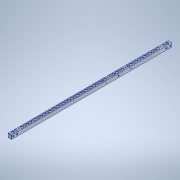
# Autodesk Inventor part: ロボットベース15x15_1
Saved by Autodesk Inventor 2020.3 (Build 243373000, 373)
## iProperties
Created: 2020-07-04
Part Number: ロボットベース15x15_1
Material: アルミニウム 6061
Document SubType Name: Modeling
Designer: totot
Density: 2.7 g/cm^3
Appearance: アルミニウム - フラット
Mass: 89.7951 g
Surface Area: 597.989 cm^2
Volume: 33.2574 cm^3
Author: totot
Autodesk Inventor part; units mm, degrees
ref_plane "YZ Plane" through (0, 0, 0) normal (1, 0, 0) x (0, 1, 0)
ref_plane "XZ Plane" through (0, 0, 0) normal (0, 1, 0) x (-1, 0, 0)
ref_plane "XY Plane" through (0, 0, 0) normal (0, 0, 1) x (1, 0, 0)
sketch "スケッチ1" plane through (0, 0, 0) normal (0, 0, 1) x (1, 0, 0)
  line L0 (0, 0) -> (-15, 0)
  line L1 (-15, 0) -> (-15, -15)
  line L2 (-15, -15) -> (0, -15)
  line L3 (0, -15) -> (0, 0)
  line L4 (-13.8, -1.2) -> (-1.2, -1.2)
  line L5 (-1.2, -1.2) -> (-1.2, -13.8)
  line L6 (-1.2, -13.8) -> (-13.8, -13.8)
  line L7 (-13.8, -13.8) -> (-13.8, -1.2)
  dimension "d0" = 15
  dimension "d1" = 15
  dimension "d2" = 1.2
  dimension "d3" = 1.2
  dimension "d4" = 1.2
  dimension "d5" = 1.2
  constraints: 16 end point, 4 parallel, 2 horizontal, 2 perpendicular
  measures "d0" distance of L2.end L1.end
  measures "d1" distance of L1.end L0.end
  measures "d2" distance between parallel lines of L1 L7
  measures "d3" distance between parallel lines of L4 L0
  measures "d4" distance between parallel lines of L2 L6
  measures "d5" distance between parallel lines of L5 L3
extrude "押し出し1" add sketch "スケッチ1" along normal blind 655
sketch "スケッチ2" plane through (0, -15, 0) normal (1, 0, 0) x (0, 0, -1)
  line L0 (-655, 0) -> (-655, 15) projected
  line L1 (0, 15) -> (-655, 15) projected
  line L2 (0, 0) -> (0, 15) projected
  point P0 (-7.5, 7.5)
  point P1 (-647.5, 7.5)
  dimension "d8" = 7.5
  dimension "d9" = 7.5
  dimension "d10" = 7.5
  dimension "d11" = 7.5
  measures "d8" distance from line of point (-647.5, 7.5) L0
  measures "d9" distance from line of point (-647.5, 7.5) L1
  measures "d10" distance from line of point (-7.5, 7.5) L1
  measures "d11" distance from line of point (-7.5, 7.5) L2
hole "穴1" at (0, -7.5, 7.5) at (0, -7.5, 647.5) direction (-1, 0, 0) diameter 5 end through all
sketch "スケッチ3" plane through (-15, -15, 0) normal (-1, 0, 0) x (0, 0, 1)
  line L0 (0, 0) -> (655, 0) projected
  circle A0 centre (7.5, 7.5) radius 2.5 projected
  circle A1 centre (647.5, 7.5) radius 2.5 projected
  point P0 (0, 15)
  point P1 (22.5, 7.5)
  point P2 (632.5, 7.5)
  dimension "d19" = 7.5
  dimension "d20" = 15
  dimension "d21" = 7.5
  dimension "d22" = 15
  measures "d19" distance from line of point (22.5, 7.5) L0
  measures "d20" distance of point (22.5, 7.5) A0.centre
  measures "d21" distance from line of L0 point (632.5, 7.5)
  measures "d22" distance of point (632.5, 7.5) A1.centre
hole "穴2" at (-15, -7.5, 22.5) at (-15, -7.5, 632.5) direction (1, 0, 0) diameter 3 depth 5 tip angle 118
sketch "スケッチ4" plane through (-1.2, -13.8, 0) normal (-1, 0, 0) x (0, 0, 1)
  circle A0 centre (22.5, 6.3) radius 1.5 projected
  circle A1 centre (632.5, 6.3) radius 1.5 projected
  point P0 (0, 13.8)
  constraints: 2 coincident
hole "穴3" at (-1.2, -7.5, 22.5) at (-1.2, -7.5, 632.5) direction (1, 0, 0) diameter 6 end through all
sketch "スケッチ6" plane through (-15, 0, 0) normal (0, 1, 0) x (1, 0, 0)
  line L0 (15, -655) -> (0, -655) projected
  line L1 (15, 0) -> (15, -655) projected
  line L2 (15, 0) -> (0, 0) projected
  point P0 (7.5, -37.5)
  point P1 (7.5, -617.5)
  dimension "d37" = 37.5
  dimension "d38" = 7.5
  dimension "d39" = 7.5
  dimension "d40" = 37.5
  measures "d37" distance from line of point (7.5, -617.5) L0
  measures "d38" distance from line of point (7.5, -617.5) L1
  measures "d39" distance from line of point (7.5, -37.5) L1
  measures "d40" distance from line of point (7.5, -37.5) L2
hole "穴4" at (-7.5, 0, 37.5) at (-7.5, 0, 617.5) direction (0, -1, 0) diameter 3 end through all
sketch "スケッチ7" plane through (-15, -15, 0) normal (-1, 0, 0) x (0, 0, 1)
  line L0 (0, 15) -> (655, 15) projected
  line L1 (0, 15) -> (0, 0) projected
  point P0 (218.3333, 7.5)
  dimension "d59" = 655
  dimension "d60" = 218.3333
  dimension "d61" = 7.5
  measures "d59" distance of L0.start L0.end
  measures "d60" distance from line of point (218.333, 7.5) L1
  measures "d61" distance from line of point (218.333, 7.5) L0
hole "穴5" at (-15, -7.5, 218.3333) direction (1, 0, 0) diameter 5 end through all
sketch "スケッチ8" plane through (-15, -15, 0) normal (-1, 0, 0) x (0, 0, 1)
  line L0 (0, 15) -> (655, 15) projected
  circle A0 centre (218.3333, 7.5) radius 2.5 projected
  point P0 (167.8333, 7.5)
  point P1 (268.8333, 7.5)
  dimension "d62" = 7.5
  dimension "d63" = 7.5
  dimension "d64" = 101
  dimension "d65" = 50.5
  measures "d62" distance from line of point (167.833, 7.5) L0
  measures "d63" distance from line of point (268.833, 7.5) L0
  measures "d64" distance of point (268.833, 7.5) point (167.833, 7.5)
  measures "d65" distance of point (167.833, 7.5) A0.centre
hole "穴6" at (-15, -7.5, 167.8333) at (-15, -7.5, 268.8333) direction (1, 0, 0) diameter 3 end through all
sketch "スケッチ9" plane through (-15, 0, 0) normal (0, 1, 0) x (1, 0, 0)
  line L0 (15, 0) -> (15, -655) projected
  line L1 (15, 0) -> (0, 0) projected
  point P0 (7.5, -182.8333)
  point P1 (7.5, -253.8333)
  point P2 (9.8445, -218.3333)
  dimension "d73" = 7.5
  dimension "d74" = 7.5
  dimension "d75" = 71
  dimension "d76" = 655
  dimension "d85" = 218.3333
  dimension "d86" = 35.5
  measures "d73" distance from line of point (7.5, -182.833) L0
  measures "d74" distance from line of point (7.5, -253.833) L0
  measures "d75" distance of point (7.5, -182.833) point (7.5, -253.833)
  measures "d76" distance of L0.start L0.end
  measures "d85" distance from line of L1 point (9.844, -218.333)
  measures "d86" vertical distance of point (9.844, -218.333) point (7.5, -253.833)
hole "穴7" at (-7.5, 0, 182.8333) at (-7.5, 0, 253.8333) direction (0, -1, 0) diameter 3 end through all
sketch "スケッチ10" plane through (-15, -15, 0) normal (0, -1, 0) x (1, 0, 0)
  circle A0 centre (7.5, 37.5) radius 1.5 projected
  line L0 (0, 0) -> (15, 0) projected
  line L1 (0, 0) -> (0, 655) projected
  line L2 (0, 655) -> (15, 655) projected
  circle A1 centre (7.5, 182.8333) radius 1.5 projected
  circle A2 centre (7.5, 253.8333) radius 1.5 projected
  circle A3 centre (7.5, 617.5) radius 1.5 projected
  point P0 (7.5, 12.5)
  point P1 (7.5, 25)
  point P2 (7.5, 630)
  point P3 (7.5, 642.5)
  point P4 (7.5, 48.6795)
  point P5 (7.5, 194.6667)
  point P6 (7.5, 206.5)
  point P7 (7.5, 218.3333)
  point P8 (7.5, 230.1667)
  point P9 (7.5, 242)
  point P10 (7.5, 59.859)
  point P11 (7.5, 71.0385)
  point P12 (7.5, 82.2179)
  point P13 (7.5, 93.3974)
  point P14 (7.5, 104.5769)
  point P15 (7.5, 115.7564)
  point P16 (7.5, 126.9359)
  point P17 (7.5, 138.1154)
  point P18 (7.5, 149.2949)
  point P19 (7.5, 160.4744)
  point P20 (7.5, 171.6538)
  point P21 (7.5, 265.1979)
  point P22 (7.5, 276.5625)
  point P23 (7.5, 287.9271)
  point P24 (7.5, 299.2917)
  point P25 (7.5, 310.6562)
  point P26 (7.5, 322.0208)
  point P27 (7.5, 333.3854)
  point P28 (7.5, 344.75)
  point P29 (7.5, 356.1146)
  point P30 (7.5, 367.4792)
  point P31 (7.5, 378.8438)
  point P32 (7.5, 390.2083)
  point P33 (7.5, 401.5729)
  point P34 (7.5, 412.9375)
  point P35 (7.5, 424.3021)
  point P36 (7.5, 435.6667)
  point P37 (7.5, 447.0312)
  point P38 (7.5, 458.3958)
  point P39 (7.5, 469.7604)
  point P40 (7.5, 481.125)
  point P41 (7.5, 492.4896)
  point P42 (7.5, 503.8542)
  point P43 (7.5, 515.2188)
  point P44 (7.5, 526.5833)
  point P45 (7.5, 537.9479)
  point P46 (7.5, 549.3125)
  point P47 (7.5, 560.6771)
  point P48 (7.5, 572.0417)
  point P49 (7.5, 583.4062)
  point P50 (7.5, 594.7708)
  point P51 (7.5, 606.1354)
  dimension "d87" = 37.5
  dimension "d88" = 7.5
  dimension "d89" = 7.5
  dimension "d90" = 12.5
  dimension "d91" = 12.5
  dimension "d92" = 7.5
  dimension "d93" = 7.5
  dimension "d94" = 12.5
  dimension "d95" = 12.5
  dimension "d96" = 7.5
  dimension "d97" = 145.3333
  dimension "d98" = 71
  dimension "d101" = 11.8333
  dimension "d106" = 7.5
  dimension "d107" = 11.8333
  dimension "d108" = 11.1795
  dimension "d111" = 11.1795
  dimension "d116" = 363.6667
  dimension "d117" = 11.3646
  dimension "d118" = 7.5
  dimension "d121" = 11.3646
  constraints: 3 vertical, 45 other
  measures "d87" distance from line of A0.centre L0
  measures "d88" distance from line of point (7.5, 25) L1
  measures "d89" distance from line of point (7.5, 12.5) L1
  measures "d90" distance from line of point (7.5, 12.5) L0
  measures "d91" distance of point (7.5, 25) point (7.5, 12.5)
  measures "d92" distance from line of point (7.5, 630) L1
  measures "d93" distance from line of point (7.5, 642.5) L1
  measures "d94" distance of point (7.5, 630) point (7.5, 642.5)
  measures "d95" distance from line of point (7.5, 642.5) L2
  measures "d96" distance from line of point (7.5, 194.667) L1
  measures "d97" distance of A1.centre A0.centre
  measures "d98" distance of A2.centre A1.centre
  measures "d101" distance of point (7.5, 194.667) point (7.5, 206.5)
  measures "d106" distance from line of point (7.5, 48.679) L1
  measures "d107" distance of A1.centre point (7.5, 194.667)
  measures "d108" distance of point (7.5, 48.679) A0.centre
  measures "d111" distance of point (7.5, 48.679) point (7.5, 59.859)
  measures "d116" distance of A3.centre A2.centre
  measures "d117" distance of point (7.5, 265.198) A2.centre
  measures "d118" distance from line of point (7.5, 265.198) L1
  measures "d121" distance of point (7.5, 265.198) point (7.5, 276.562)
hole "穴8" at (-7.5, -15, 12.5) at (-7.5, -15, 25) at (-7.5, -15, 630) at (-7.5, -15, 642.5) at (-7.5, -15, 48.6795) at (-7.5, -15, 194.6667) at (-7.5, -15, 206.5) at (-7.5, -15, 218.3333) at (-7.5, -15, 230.1667) at (-7.5, -15, 242) at (-7.5, -15, 59.859) at (-7.5, -15, 71.0385) at (-7.5, -15, 82.2179) at (-7.5, -15, 93.3974) at (-7.5, -15, 104.5769) at (-7.5, -15, 115.7564) at (-7.5, -15, 126.9359) at (-7.5, -15, 138.1154) at (-7.5, -15, 149.2949) at (-7.5, -15, 160.4744) at (-7.5, -15, 171.6538) at (-7.5, -15, 265.1979) at (-7.5, -15, 276.5625) at (-7.5, -15, 287.9271) at (-7.5, -15, 299.2917) at (-7.5, -15, 310.6562) at (-7.5, -15, 322.0208) at (-7.5, -15, 333.3854) at (-7.5, -15, 344.75) at (-7.5, -15, 356.1146) at (-7.5, -15, 367.4792) at (-7.5, -15, 378.8438) at (-7.5, -15, 390.2083) at (-7.5, -15, 401.5729) at (-7.5, -15, 412.9375) at (-7.5, -15, 424.3021) at (-7.5, -15, 435.6667) at (-7.5, -15, 447.0312) at (-7.5, -15, 458.3958) at (-7.5, -15, 469.7604) at (-7.5, -15, 481.125) at (-7.5, -15, 492.4896) at (-7.5, -15, 503.8542) at (-7.5, -15, 515.2188) at (-7.5, -15, 526.5833) at (-7.5, -15, 537.9479) at (-7.5, -15, 549.3125) at (-7.5, -15, 560.6771) at (-7.5, -15, 572.0417) at (-7.5, -15, 583.4062) direction (0, 1, 0) diameter 10 end through all and at (-7.5, -15, 594.7708) (-7.5, -15, 606.1354)
equation "\"d3\" = d2"
equation "\"d4\" = d3"
equation "\"d5\" = d2"
equation "\"d9\" = d8"
equation "\"d11\" = d10"
equation "\"d60\" = 0.333333 * d59"
equation "\"d61\" = d57"
equation "\"d63\" = d62"
equation "\"d74\" = d73"
equation "\"d85\" = 0.333333 * d76"
equation "\"d86\" = 0.5 * d75"
equation "\"d89\" = d88"
equation "\"d90\" = 0.333333 * d87"
equation "\"d91\" = d90"
equation "\"d94\" = d91"
equation "\"d95\" = d94"
equation "\"d101\" = 0.166667 * d98"
equation "\"d106\" = d88"
equation "\"d107\" = d101"
equation "\"d108\" = 0.0769231 * d97"
equation "\"d111\" = d108"
equation "\"d117\" = 0.03125 * d116"
equation "\"d121\" = d117"
equation "\"d57\" = 7.5"
